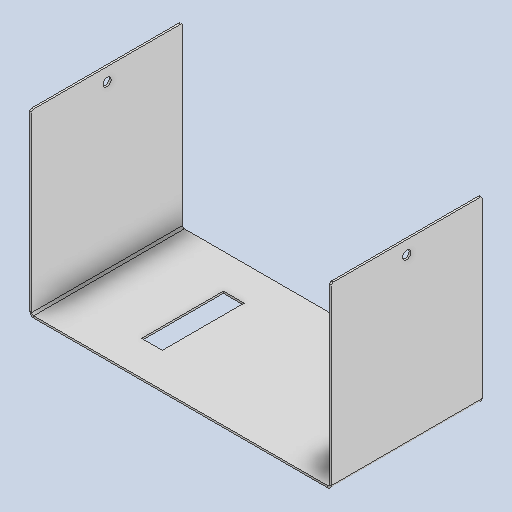
# Autodesk Inventor part: metal_cap_fixed
Saved by Autodesk Inventor 2022 (Build 260153000, 153)
## iProperties
Created: 2024-12-12
Part Number: metal_cap_fixed
Material: Типовые
Document SubType Name: Sheet Metal
Designer: Andrey
Density: 1 g/cm^3
Sheet Metal Rule: По умолчанию_мм
Appearance: По умолчанию
Flat Pattern Width: 4 cm
Flat Pattern Length: 17.3262 cm
Flat Pattern Area: 69.3048 cm^2
Sheet Metal Width: 40,000 мм
Sheet Metal Length: 173,262 мм
Sheet Metal Area: 6930,478 мм^2
Author: Andrey
Autodesk Inventor part; units mm, degrees
ref_plane "YZ Plane" through (0, 0, 0) normal (1, 0, 0) x (0, 1, 0)
ref_plane "XZ Plane" through (0, 0, 0) normal (0, 1, 0) x (-1, 0, 0)
ref_plane "XY Plane" through (0, 0, 0) normal (0, 0, 1) x (1, 0, 0)
sketch "Эскиз1" plane through (0, 0, 0) normal (0, 1, 0) x (-1, 0, 0)
  line L0 (19.5, 10.85) -> (19.5, -10.85)
  line L1 (19.5, -10.85) -> (14, -10.85)
  line L2 (14, -10.85) -> (14, 10.85)
  line L3 (14, 10.85) -> (19.5, 10.85)
  line L4 (39, -20) -> (39, 20)
  line L5 (-39, 20) -> (39, 20)
  line L6 (-39, 20) -> (-39, -20)
  line L7 (39, -20) -> (-39, -20)
  line L8 (-40, -20) -> (-40, 20)
  line L9 (-40, -20) -> (-39, -20)
  line L10 (-39, 20) -> (-40, 20)
  line L11 (39, -20) -> (40, -20)
  line L12 (40, 20) -> (40, -20)
  line L13 (40, 20) -> (39, 20)
  point P0 (0, 0)
  point P1 (0, 0)
extrude "Пластина1" add sketch "Эскиз1" along normal blind 0.5
sketch "Эскиз2" plane through (39.5, 0, -20) normal (1, 0, 0) x (0, 1, 0)
  line L0 (0, 40) -> (0, 0)
  line L1 (0, 0) -> (47.5, 0)
  line L2 (47.5, 0) -> (47.5, 40)
  line L3 (47.5, 40) -> (0, 40)
  constraints: 6 end point, 1 horizontal, 1 perpendicular, 1 vertical
edge flange "Фланец1" height 47.5 angle 90 thickness 0.5 bend radius 0.5 thickness toward (1, 0, 0) relief straight relief width 0.5 relief depth 0.25 corner gap 0.5 corner form 0 edges at (40, 0.5, 0) (-40, 0.5, 0) wall of the first edge with corners at (39.5, 0, 20) (39.5, 0, -20) (39.5, 47.5, -20) (39.5, 47.5, 20)
bend "Сгиб1"
corner "УглСтык1"
sketch "Эскиз3" plane through (40, 47.5, 20) normal (1, 0, 0) x (0, 0, -1)
  circle A0 centre (20, 43) radius 1.1
  arc A1 (40, 46) -> (39.5, 46.5) centre (39.5, 46) ccw
  line L0 (0.5, 46.5) -> (39.5, 46.5)
  arc A2 (0.5, 46.5) -> (0, 46) centre (0.5, 46) ccw
  line L1 (0, 0) -> (0, 46)
  line L2 (0, 0) -> (40, 0)
  line L3 (40, 46) -> (40, 0)
  line L4 (0, -46.5) -> (40, -46.5) projected
  line L5 (40, 0) -> (40, -46.5) projected
  line L6 (0, 0) -> (40, 0) projected
  line L7 (0, -46.5) -> (0, 0) projected
  circle A3 centre (20, -3.5) radius 1.1
  arc A4 (40, -0.5) -> (39.5, 0) centre (39.5, -0.5) ccw
  line L8 (0.5, 0) -> (39.5, 0)
  arc A5 (0.5, 0) -> (0, -0.5) centre (0.5, -0.5) ccw
  line L9 (0, -46.5) -> (0, -0.5)
  line L10 (0, -46.5) -> (40, -46.5)
  line L11 (40, -0.5) -> (40, -46.5)
  point P0 (20, -47.5)
  point P1 (20, 23)
  point P2 (20, -23.5)
  constraints: 16 end point, 8 point on circle, 6 centre point
extrude "Вырез1" cut sketch "Эскиз3" against normal blind 90 contours L5 A4 L2 | A5 L7 L2 | A3
equation "\"d0\" = Толщина"
equation "\"d1\" = Ширина_просечки"
equation "\"d2\" = Глубина_просечки"
equation "\"d3\" = Мин_остаток"
equation "\"d4\" = Радиус_перехода"
equation "\"d7\" = Радиус_гибки"
equation "\"d8\" = Размер_просечки"
equation "\"d9\" = Размер_зазора"
equation "\"d10\" = Радиус_Якоби"
equation "\"Радиус_гибки\" = Толщина"
equation "\"Ширина_просечки\" = Толщина"
equation "\"Глубина_просечки\" = 0.5 * Толщина"
equation "\"Размер_просечки\" = 4 * Толщина"
equation "\"Мин_остаток\" = 2 * Толщина"
equation "\"Радиус_перехода\" = Радиус_гибки"
equation "\"Радиус_Якоби\" = Радиус_гибки"
equation "\"Размер_зазора\" = Толщина"
equation "\"Толщина\" = 0.5"
